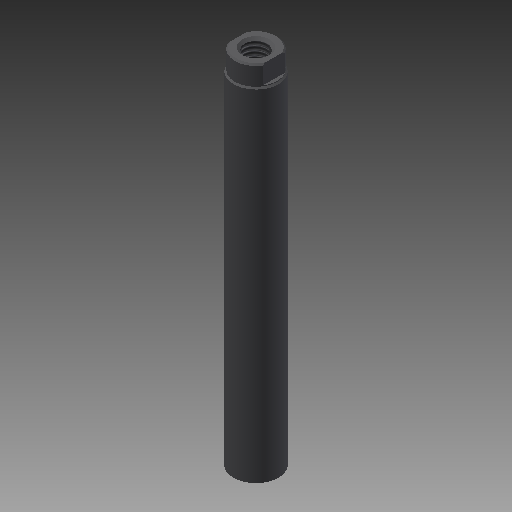
# Autodesk Inventor part: FO-042.5112.511-00_rod
Saved by Autodesk Inventor 2017 (Build 210142000, 142)
## iProperties
Category: PARTsolutions
Company: BIMBA
Created: 2017-01-25
Part Number: FO-042.5112.511-00_rod
Catalog Web Link: www.cadenas.de
Description: FO1 Basic Model Rod-Bimba FLAT-1
Vendor: BIMBA
Document SubType Name: Modeling
Designer: psAdmin
Manufacturer: BIMBA
Mass: 2.95863 g
Surface Area: 18.3643 cm^2
Volume: 2.95863 cm^3
Density: 1 g/cm^3
Material: Generic
Appearance: PSOLRGB-180-180-180
PSOL_IDENT_0: {$CADENAS_DATA\23d-libs\bimba\bimba\bimba_imperial\bimba_full_line\flat_cylinders\fo1\fo1_basic_mode
PSOL_IDENT_1: l_rod.prj},229 {VTYP=3D},{NB=FO-042.5112.511-00_rod},{LINA=FO-042.5112.511-00_rod},{NN=FO1 Basic Mod
PSOL_IDENT_2: el Rod},{DATE=01.12.2016 06:16:11},{GEOMDATE=02.11.2016 11:55:39},{VERSION=},{LINEID=20},{LINESUBID=
PSOL_IDENT_3: -1},{WBVAR=STROKE,LENGTH,ER,RT,HR,FCD,RCD}  {NB=FO-042.5112.511-00_rod},{LINA=FO-042.5112.511-00_rod
PSOL_IDENT_4: },{KT=DUMMY},{PN=FO-042.5112.511-00},{BORE=0.75000000},{BOREPN=04},{STROKE=2.51100},{STROKEMIN=0.46}
PSOL_IDENT_5: ,{LENGTHALG=2.511},{LENGTH=2.51100},{ER=},{RT=},{HR=},{HRALG='','N/A'},{EE=},{EEALG='','Without Extr
PSOL_IDENT_6: a Extension','EE','With Extra Extension'},{EELALG=0},{EELMAX=17.489},{EEL=0},{EELPN=},{A=1.50000000}
PSOL_IDENT_7: ,{BA=0.56000},{BB=0.69000},{BC=1.94},{BD=2.19},{C=1.22000000},{DD=4.00000000},{D=0.13800000},{CPIL=0
PSOL_IDENT_8: .15600000},{DC=0.23500000},{DCP=0.14800000},{DCD=1.21800000},{ES=0.19000000},{EC=0.19000000},{ED=0.4
PSOL_IDENT_9: 6000000},{F=0.31250000},{H=0.24750000},{J=0.34000000},{K=0.14000000},{L=0.19000000},{LDP=0.12600000}
PSOL_IDENT_10: ,{LP=0.12500000},{LPDP=0.44000000},{TD=0.80500000},{TDDP=0.17000},{TD1=0.80000},{TD2=0.81200},{TDIN=
PSOL_IDENT_11: 0.75000},{LSF=0.31250000},{LSFDP=0.02000000},{BC1=0.81000},{BC2=1.38000},{BC3=1.94000},{BC4=2.50000}
PSOL_IDENT_12: ,{BD1=1.06000},{BD2=1.62000},{BD3=2.19000},{BD4=2.75000},{MT=0.19000000},{CMT=0.19000000},{LG=0.3750
PSOL_IDENT_13: 0000},{HF=0.14000000},{HM=0.09000000},{HD=0.14},{HALG=0},{HDY=0.46},{HDH=1.591},{LG1=0.00000000},{FC
PSOL_IDENT_14: D=0},{RCD=0},{NPT=0.000},{FTL1=0.460},{FTLSR=0.000},{TDD=0.554},{TDDSR=0.000},{TDDSRC=0.000},{TDDC=0
PSOL_IDENT_15: .585},{NPTTDD=0.000},{FTL=0.460},{TDDR=0.554},{TDDRC=0.585},{WD=0.293},{TL=0.135},{HRID=0.140},{HRNT
PSOL_IDENT_16: P=0.000},{HRMT=0.093},{GL=0.050},{GD=0.141},{GR=0.019},{GLC=0.066},{GDC=0.126},{GRC=0.034},{NR=1.000
PSOL_IDENT_17: },{RTALG='', 'Standard', 'CFT', 'Coarse Female Thread', 'CMT'  , 'Male Rod Thread (Coarse)','MT', 'M
PSOL_IDENT_18: ale Rod End (Fine)', 'NT'  , 'Non-Threaded Rod'}
NN: FO1 Basic Model Rod
NT: Bimba FLAT-1
NB: FO-042.5112.511-00_rod
NBSYN: $PN._rod
LINA: FO-042.5112.511-00_rod
PN: FO-042.5112.511-00
BORE: 3/4
BOREPN: 04
STROKE: 2.51100
LENGTH: 2.51100
ER: Single End Rod
RT: Standard
HR: N/A
A: 1.50000000
BA: 0.56000
BB: 0.69000
C: 1.22000000
DD: 4.00000000
D: 0.13800000
CPIL: 0.15600000
DC: 0.23500000
DCP: 0.14800000
DCD: 1.21800000
ES: 0.19000000
EC: 0.19000000
ED: 0.46000000
F: 0.31250000
H: 0.24750000
J: 0.34000000
K: 0.14000000
L: 0.19000000
LDP: 0.12600000
LP: 0.12500000
LPDP: 0.44000000
TD: 0.80500000
TDDP: 0.17000
TD1: 0.80000
TD2: 0.81200
TDIN: 0.75000
LSF: 0.31250000
LSFDP: 0.02000000
BC1: 0.81000
BC2: 1.38000
BC3: 1.94000
BC4: 2.50000
BD1: 1.06000
BD2: 1.62000
BD3: 2.19000
BD4: 2.75000
MT: 0.19000000
CMT: 0.19000000
LG: 0.37500000
HF: 0.14000000
HM: 0.09000000
FCD: 0
RCD: 0
NPT: 0.000
FTL1: 0.460
FTLSR: 0.000
TDD: 0.554
TDDSR: 0.000
TDDSRC: 0.000
TDDC: 0.585
NPTTDD: 0.000
WD: 0.293
TL: 0.135
HRID: 0.140
HRNTP: 0.000
HRMT: 0.093
GL: 0.050
GD: 0.141
GR: 0.019
GLC: 0.066
GDC: 0.126
GRC: 0.034
NR: 1.000
SUPPLIER: BIMBA
ARTICLENO: FO-042.5112.511-00_rod
BOMINFO: FO-042.5112.511-00_rod
CREATOR: CADENAS GmbH
Title: FO-042.5112.511-00_rod
Author: Cadenas PARTsolutions
Comments: Bimba FLAT-1
Autodesk Inventor part; units mm, degrees
sketch "Sketch_31" plane through (0, 0, 0) normal (0, 0, 1) x (1, 0, 0)
  line L0 (0, 0) -> (0, 63.7794)
  line L1 (0, 63.7794) -> (3.473, 63.7794)
  line L2 (3.473, 63.7794) -> (3.7211, 63.5313)
  line L3 (3.7211, 63.5313) -> (3.7211, 60.3504)
  line L4 (3.7211, 60.3504) -> (3.9688, 60.1028)
  line L5 (3.9688, 60.1028) -> (3.9688, 0)
  line L6 (3.9688, 0) -> (0, 0)
  line L7 (0, 0) -> (0, 63.7794)
  constraints: 16 end point
revolve "Revolution1" add sketch "Sketch_31" angle 360 about axis through (0, 0, 0) along (0, -1, 0)
sketch "Sketch2" plane through (0, 63.7794, 0) normal (0, 1, 0) x (1, 0, 0)
  point P0 (0, 0)
hole "Hole1" at (0, 63.7794, 0) direction (0, -1, 0) diameter 3.9624 depth 12.9263 tip angle 120 countersink diameter 4.826 countersink angle 90 thread size "10-32 UNF" class "2B" standard "ANSI Unified Screw Threads"
sketch "Sketch_29" plane through (0, 63.7794, 0) normal (0, 1, 0) x (1, 0, 0)
  line L0 (-6.2865, -15.875) -> (6.2865, -15.875)
  line L1 (6.2865, -15.875) -> (6.2865, 15.875)
  line L2 (6.2865, 15.875) -> (-6.2865, 15.875)
  line L3 (-6.2865, 15.875) -> (-6.2865, -15.875)
  line L4 (-3.1433, -7.9375) -> (3.1433, -7.9375)
  line L5 (3.1433, -7.9375) -> (3.1433, 7.9375)
  line L6 (3.1433, 7.9375) -> (-3.1433, 7.9375)
  line L7 (-3.1433, 7.9375) -> (-3.1433, -7.9375)
  constraints: 16 end point
extrude "Extrusion1" cut sketch "Sketch_29" against normal blind 3.302
ref_plane "b11_XY" through (0, 0, 0) normal (0, 1, 0) x (1, 0, 0)
ref_plane "b11_YZ" through (0, 0, 0) normal (1, 0, 0) x (0, 0, -1)
ref_plane "b11_ZX" through (0, 0, 0) normal (0, 0, -1) x (0, 1, 0)
ref_plane "b2_XY" through (0, 63.7794, 0) normal (0, 1, 0) x (1, 0, 0)
ref_plane "b2_YZ" through (0, 63.7794, 0) normal (1, 0, 0) x (0, 0, -1)
ref_plane "b2_ZX" through (0, 63.7794, 0) normal (0, 0, -1) x (0, 1, 0)
ref_plane "f1_XY" through (0, 63.7794, 3.9688) normal (1, 0, 0) x (0, 0, -1)
ref_plane "f1_YZ" through (0, 63.7794, 3.9688) normal (0, 0, -1) x (0, 1, 0)
ref_plane "f1_ZX" through (0, 63.7794, 3.9688) normal (0, 1, 0) x (1, 0, 0)
ref_plane "f2_XY" through (0, 63.7794, -3.9688) normal (1, 0, 0) x (0, 0, -1)
ref_plane "f2_YZ" through (0, 63.7794, -3.9688) normal (0, 0, -1) x (0, 1, 0)
ref_plane "f2_ZX" through (0, 63.7794, -3.9688) normal (0, 1, 0) x (1, 0, 0)
ref_plane "h1_XY" through (-3.1433, 63.7794, 0) normal (0, 1, 0) x (1, 0, 0)
ref_plane "h1_YZ" through (-3.1433, 63.7794, 0) normal (1, 0, 0) x (0, 0, -1)
ref_plane "h1_ZX" through (-3.1433, 63.7794, 0) normal (0, 0, -1) x (0, 1, 0)
ref_plane "h2_XY" through (3.1433, 63.7794, 0) normal (0, 1, 0) x (1, 0, 0)
ref_plane "h2_YZ" through (3.1433, 63.7794, 0) normal (1, 0, 0) x (0, 0, -1)
ref_plane "h2_ZX" through (3.1433, 63.7794, 0) normal (0, 0, -1) x (0, 1, 0)
ref_plane "npt1_XY" through (0, 63.7794, 0) normal (0, 1, 0) x (1, 0, 0)
ref_plane "npt1_YZ" through (0, 63.7794, 0) normal (1, 0, 0) x (0, 0, -1)
ref_plane "npt1_ZX" through (0, 63.7794, 0) normal (0, 0, -1) x (0, 1, 0)
ref_plane "npt2_XY" through (0, 63.7794, 0) normal (0, 1, 0) x (1, 0, 0)
ref_plane "npt2_YZ" through (0, 63.7794, 0) normal (1, 0, 0) x (0, 0, -1)
ref_plane "npt2_ZX" through (0, 63.7794, 0) normal (0, 0, -1) x (0, 1, 0)
ref_plane "rod_XY" through (0, 63.7794, 0) normal (0, 1, 0) x (1, 0, 0)
ref_plane "rod_YZ" through (0, 63.7794, 0) normal (1, 0, 0) x (0, 0, -1)
ref_plane "rod_ZX" through (0, 63.7794, 0) normal (0, 0, -1) x (0, 1, 0)
ref_plane "rod_to_part_XY" through (0, 0, 0) normal (0, 1, 0) x (1, 0, 0)
ref_plane "rod_to_part_YZ" through (0, 0, 0) normal (1, 0, 0) x (0, 0, -1)
ref_plane "rod_to_part_ZX" through (0, 0, 0) normal (0, 0, -1) x (0, 1, 0)
ref_plane "th1_XY" through (0, 63.7794, 2.413) normal (0, 1, 0) x (1, 0, 0)
ref_plane "th1_YZ" through (0, 63.7794, 2.413) normal (1, 0, 0) x (0, 0, -1)
ref_plane "th1_ZX" through (0, 63.7794, 2.413) normal (0, 0, -1) x (0, 1, 0)
ref_plane "th2_XY" through (0, 63.7794, -2.413) normal (0, 1, 0) x (1, 0, 0)
ref_plane "th2_YZ" through (0, 63.7794, -2.413) normal (1, 0, 0) x (0, 0, -1)
ref_plane "th2_ZX" through (0, 63.7794, -2.413) normal (0, 0, -1) x (0, 1, 0)
ref_plane "to_rod_pivot_XY" through (0, 63.7794, 0) normal (0, 1, 0) x (1, 0, 0)
ref_plane "to_rod_pivot_YZ" through (0, 63.7794, 0) normal (1, 0, 0) x (0, 0, -1)
ref_plane "to_rod_pivot_ZX" through (0, 63.7794, 0) normal (0, 0, -1) x (0, 1, 0)
ref_plane "to_rod_pivot1_XY" through (0, 0, 0) normal (0, 1, 0) x (1, 0, 0)
ref_plane "to_rod_pivot1_YZ" through (0, 0, 0) normal (1, 0, 0) x (0, 0, -1)
ref_plane "to_rod_pivot1_ZX" through (0, 0, 0) normal (0, 0, -1) x (0, 1, 0)
body "Solid1"
